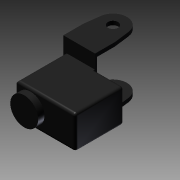
# Autodesk Inventor part: Wrist
Saved by Autodesk Inventor 2012 (Build 160160000, 160)
## iProperties
Created: 2013-02-21
Part Number: Wrist
Material: Default
Document SubType Name: Modeling
Designer: Andrew
Density: 1 g/cm^3
Author: Andrew
Autodesk Inventor part; units mm, degrees
ref_plane "YZ Plane" through (0, 0, 0) normal (1, 0, 0) x (0, 1, 0)
ref_plane "XZ Plane" through (0, 0, 0) normal (0, 1, 0) x (-1, 0, 0)
ref_plane "XY Plane" through (0, 0, 0) normal (0, 0, 1) x (1, 0, 0)
sketch "Sketch1" plane through (0, 0, 0) normal (0, 0, 1) x (1, 0, 0)
  line L0 (5.75, 38.85) -> (2.7639, 38.85)
  arc A0 (2.7639, 38.85) -> (0.767, 36.9611) centre (2.7639, 36.85) ccw
  arc A1 (0.767, 36.9611) -> (0.75, 36.35) centre (11.75, 36.35) ccw
  line L1 (0.75, 7.85) -> (0.75, 36.35)
  line L2 (22.75, 7.85) -> (0.75, 7.85)
  line L3 (22.75, 7.85) -> (22.75, 36.35)
  arc A2 (22.75, 36.35) -> (22.733, 36.9611) centre (11.75, 36.35) ccw
  arc A3 (22.733, 36.9611) -> (20.7361, 38.85) centre (20.7361, 36.85) ccw
  line L4 (20.7361, 38.85) -> (17.75, 38.85)
  arc A4 (17.75, 38.85) -> (15.75, 36.85) centre (17.75, 36.85) ccw
  line L5 (15.75, 36.85) -> (15.75, 36.35)
  arc A5 (7.75, 36.35) -> (15.75, 36.35) centre (11.75, 36.35) ccw
  line L6 (7.75, 36.85) -> (7.75, 36.35)
  arc A6 (7.75, 36.85) -> (5.75, 38.85) centre (5.75, 36.85) ccw
  line L7 (6.75, 13.35) -> (6.75, 15.35)
  arc A7 (7.75, 16.35) -> (6.75, 15.35) centre (7.75, 15.35) ccw
  line L8 (7.75, 16.35) -> (15.75, 16.35)
  arc A8 (16.75, 15.35) -> (15.75, 16.35) centre (15.75, 15.35) ccw
  line L9 (16.75, 15.35) -> (16.75, 13.35)
  arc A9 (15.75, 12.35) -> (16.75, 13.35) centre (15.75, 13.35) ccw
  line L10 (15.75, 12.35) -> (7.75, 12.35)
  arc A10 (6.75, 13.35) -> (7.75, 12.35) centre (7.75, 13.35) ccw
  line L11 (6.75, 21.35) -> (6.75, 23.35)
  arc A11 (7.75, 24.35) -> (6.75, 23.35) centre (7.75, 23.35) ccw
  line L12 (7.75, 24.35) -> (15.75, 24.35)
  arc A12 (16.75, 23.35) -> (15.75, 24.35) centre (15.75, 23.35) ccw
  line L13 (16.75, 23.35) -> (16.75, 21.35)
  arc A13 (15.75, 20.35) -> (16.75, 21.35) centre (15.75, 21.35) ccw
  line L14 (15.75, 20.35) -> (7.75, 20.35)
  arc A14 (6.75, 21.35) -> (7.75, 20.35) centre (7.75, 21.35) ccw
  circle A15 centre (3.75, 18.35) radius 1.1
  circle A16 centre (19.75, 18.35) radius 1.1
  circle A17 centre (19.75, 36.35) radius 1
  circle A18 centre (17.4069, 30.6931) radius 1
  circle A19 centre (11.75, 28.35) radius 1
  circle A20 centre (6.0931, 30.6931) radius 1
  circle A21 centre (3.75, 36.35) radius 1
  line L15 (11.75, 7.85) -> (11.75, 6.35)
  line L16 (22.75, 7.85) -> (22.75, 6.35)
  line L17 (22.75, 6.35) -> (0.75, 6.35)
  line L18 (0.75, 6.35) -> (0.75, 7.85)
  line L19 (22.75, 6.35) -> (47, 6.35)
  line L20 (11.75, 6.35) -> (11.75, -37)
  line L21 (11.75, -37) -> (22.75, -37)
  line L22 (11.75, -37) -> (0.75, -37)
  line L23 (0.75, -37) -> (0.75, -32)
  line L24 (0.75, -32) -> (22.75, -32)
  line L25 (22.75, -32) -> (22.75, -37)
  line L26 (0.75, -32) -> (0.75, 6.35)
  line L27 (22.75, -32) -> (47, -32)
  line L28 (47, -32) -> (47, 6.35)
  dimension "d0" = 24.25
  dimension "d1" = 43.35
  dimension "d2" = 11
  dimension "d3" = 11
  dimension "d4" = 5
  constraints: 28 end point, 7 perpendicular, 4 parallel, 2 collinear, 1 midpoint
  measures "d0" distance of L16.end L19.end
  measures "d1" distance of L15.end L20.end
  measures "d2" distance of L20.end L21.end
  measures "d3" distance of L20.end L22.end
  measures "d4" distance of L22.end L23.end
extrude "Extrusion1" add sketch "Sketch1" along normal mid plane 26 contours L17 L20 L24 L26 | L17 L19 L28 L27 L24 L20
sketch "Sketch2" plane through (0.75, -32, 13) normal (0, -1, 0) x (1, 0, 0)
  circle A0 centre (11, -13) radius 11
  point P0 (-0.75, -13)
  dimension "d8" = 22
  constraints: 1 centre point
  measures "d8" diameter of A0
extrude "Extrusion2" add sketch "Sketch2" along normal blind 5
sketch "Sketch3" plane through (0.75, 6.35, 13) normal (0, 1, 0) x (1, 0, 0)
  line L0 (0, 26) -> (0, 0) projected
  line L1 (-1.5, 13) -> (-1.5, -8)
  line L2 (-1.5, -8) -> (23.5, -8)
  line L3 (23.5, -8) -> (23.5, 34)
  line L4 (23.5, 34) -> (-1.5, 34)
  line L5 (-1.5, 34) -> (-1.5, 13)
  line L6 (-1.5, 34) -> (-1.5, 37)
  line L7 (-1.5, 37) -> (23.5, 37)
  line L8 (23.5, 37) -> (23.5, 34)
  line L9 (23.5, -8) -> (23.5, -11)
  line L10 (23.5, -11) -> (-1.5, -11)
  line L11 (-1.5, -11) -> (-1.5, -8)
  line L12 (46.25, 26) -> (0, 26) projected
  line L13 (-1.5, 13) -> (-3, 13)
  point P0 (-0.75, 13)
  dimension "d13" = 21
  dimension "d14" = 25
  dimension "d15" = 42
  dimension "d16" = 3
  dimension "d17" = 3
  dimension "d30" = 1.5
  constraints: 24 end point, 5 parallel, 4 perpendicular, 2 collinear
  measures "d13" distance of L1.start L1.end
  measures "d14" distance of L1.end L2.end
  measures "d15" distance of L2.end L3.end
  measures "d16" distance of L4.end L6.end
  measures "d17" distance of L2.end L9.end
  measures "d30" distance of L1.start L13.end
extrude "Extrusion3" add sketch "Sketch3" along normal blind 1.5
sketch "Sketch4" plane through (0.75, 7.85, 13) normal (0, 1, 0) x (1, 0, 0)
  line L0 (-1.5, -11) -> (-1.5, 37) projected
  line L1 (23.5, -11) -> (-1.5, -11) projected
  line L2 (23.5, 37) -> (23.5, -11) projected
  line L3 (-1.5, 37) -> (23.5, 37) projected
  line L4 (23.5, -11) -> (23.5, -8)
  line L5 (23.5, -8) -> (-1.5, -8)
  line L6 (-1.5, 37) -> (-1.5, 34)
  line L7 (-1.5, 34) -> (23.5, 34)
  line L8 (23.5, 34) -> (23.5, 37)
  line L9 (23.5, 37) -> (-1.5, 37)
  line L10 (21.4157, -11) -> (-1.5, -11)
  line L11 (-1.5, -8) -> (-1.5, -11)
  point P0 (-0.75, 13)
  dimension "d20" = 3
  dimension "d21" = 3
  constraints: 16 end point, 5 point on line, 3 perpendicular, 2 collinear, 1 parallel
  measures "d20" distance of L1.start L4.end
  measures "d21" distance of L0.end L6.end
fillet "Fillet1" radius 2 10 edges at (47, -12.825, -13) (47, -12.825, 13) (47, -32, 0) (23.875, -32, 13) (23.875, -32, -13) (35.625, 6.35, -13) (35.625, 6.35, 13) (0.75, -12.825, -13) (0.75, -12.825, 13) (47, 6.35, 0)
extrude "Extrusion6" add sketch "Sketch4" along normal blind 45 contours L0 L5 L2 L1 | L0 L3 L2 L7
sketch "Sketch6" plane through (24.25, 6.35, -24) normal (0, 0, -1) x (-1, 0, 0)
  line L0 (0, 0) -> (0, 46.5) projected
  line L1 (25, 46.5) -> (0, 46.5) projected
  line L2 (17.4994, 5.1489) -> (25, 5.15)
  line L3 (25, 5.15) -> (25, 15.6501)
  line L4 (25, 15.6501) -> (23.4074, 28.0489)
  arc A0 (23.4074, 28.0489) -> (1.5893, 28.0448) centre (12.4986, 26.6352) ccw
  line L5 (1.5893, 28.0448) -> (0, 15.6462)
  line L6 (0, 15.6462) -> (0, 5.1462)
  line L7 (0, 5.1462) -> (7.4986, 5.1462)
  circle A1 centre (12.5, 26.65) radius 4
  line L8 (23.5, -43.35) -> (1.5, -43.35) projected
  line L9 (23.5, -38.35) -> (12.5, -38.35) projected
  line L10 (12.5, -38.35) -> (23.5, -38.35) projected
  line L11 (12.5, -38.35) -> (12.5, -38.35) projected
  line L12 (25, 5.15) -> (25, 0)
  line L13 (0, 5.1462) -> (0, 0)
  line L14 (25, 15.6501) -> (25, 46.5)
  line L15 (0, 15.6462) -> (0, 46.5)
  line L16 (0, 46.5) -> (25, 46.5)
  point P0 (24.25, -6.35)
  constraints: 22 end point, 2 centre point, 2 collinear, 2 point on circle, 1 parallel, 1 perpendicular
extrude "Extrusion7" cut sketch "Sketch6" against normal through all
body "Solid1"
